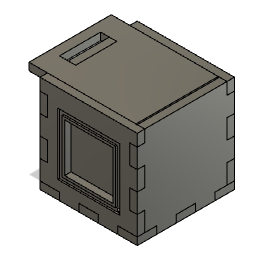
CNC Safe Box v15 (Autodesk Fusion 360 design; units mm, degrees)
Autodesk Fusion 360 part; units mm, degrees
box "BoxPrimitive1" add length 300 width 300 height 23 placed x (0, 0, -1) y (-1, 0, 0) z (0, 1, 0) at (300, 0, 0) makes body 1
sketch "Sketch3" plane through (0, 0, 0) normal (0, 0, 1) x (1, 0, 0)
  line L0 (0, 23) -> (0, 0)
  line L1 (0, 0) -> (300, 0)
  line L2 (300, 0) -> (300, 23)
  line L3 (300, 23) -> (0, 23)
  line L4 (60, 23) -> (120, 23)
  line L5 (120, 23) -> (120, 0)
  line L6 (120, 0) -> (60, 0)
  line L7 (60, 0) -> (60, 23)
  dimension "d20" = 60
  dimension "d21" = 23
  dimension "d22" = 60
  constraint horizontal L4
  constraint vertical L5
  constraint horizontal L6
  constraint vertical L7
  constraint coincident L3 L4.start
  measures "d20" distance of L4.start L4.end
  measures "d21" distance of L4.start L6.end
  measures "d22" distance of L0.start L4.start
extrude "Extrude1" cut sketch "Sketch3" against normal blind 23 contours L1 L3 L4 L5 L6 L7 bodies 1
pattern_linear "R-Pattern1" count 2 spacing 120 along (1, 0, 0) of 3 faces at (60, 7.6667, -7.6667) (80, 7.6667, -23) (120, 15.3333, -7.6667) on bodies 1
sketch "Sketch4" plane through (0, 0, 0) normal (-1, 0, 0) x (0, 0, 1)
  line L0 (-300, 23) -> (-300, 0)
  line L1 (-300, 0) -> (0, 0)
  line L2 (0, 0) -> (0, 23)
  line L3 (0, 23) -> (-300, 23)
  line L4 (-60, 23) -> (-120, 23)
  line L5 (-120, 23) -> (-120, 0)
  line L6 (-120, 0) -> (-60, 0)
  line L7 (-60, 0) -> (-60, 23)
  dimension "d29" = 60
  dimension "d30" = 23
  dimension "d31" = 60
  constraint horizontal L4
  constraint vertical L5
  constraint horizontal L6
  constraint vertical L7
  constraint coincident L3 L4.start
  measures "d29" distance of L4.start L4.end
  measures "d30" distance of L4.start L6.end
  measures "d31" distance of L2.end L4.start
extrude "Extrude2" cut sketch "Sketch4" against normal blind 23 contours L1 L3 L4 L5 L6 L7 bodies 1
pattern_linear "R-Pattern2" count 2 spacing 120 along (0, 0, -1) of 3 faces at (7.6667, 7.6667, -60) (23, 15.3333, -80) (7.6667, 15.3333, -120) on bodies 1
sketch "Sketch5" plane through (0, 0, 0) normal (0, 0, 1) x (1, 0, 0)
  line L0 (0, 0) -> (300, 0)
  line L1 (300, 0) -> (300, 300)
  line L2 (300, 300) -> (0, 300)
  line L3 (0, 300) -> (0, 0)
  dimension "d38" = 300
  dimension "d39" = 300
  constraint horizontal L0
  constraint vertical L1
  constraint horizontal L2
  constraint vertical L3
  constraint coincident L0.start L3.end
  measures "d38" distance of L0.start L0.end
  measures "d39" distance of L0.start L2.end
extrude "Extrude3" add sketch "Sketch5" against normal blind 23 separate body makes body 2
combine "Combine1" operation cut target body 2 tool bodies 1 keep tools
sketch "Sketch6" plane through (0, 0, 0) normal (-1, 0, 0) x (0, 0, 1)
  line L0 (-23, 23) -> (0, 23)
  line L1 (0, 23) -> (0, 300)
  line L2 (0, 300) -> (-23, 300)
  line L3 (-23, 300) -> (-23, 23)
  line L4 (-23, 83) -> (0, 83)
  line L5 (0, 83) -> (0, 143)
  line L6 (0, 143) -> (-23, 143)
  line L7 (-23, 143) -> (-23, 83)
  dimension "d42" = 23
  dimension "d43" = 60
  dimension "d44" = 60
  constraint horizontal L4
  constraint vertical L5
  constraint horizontal L6
  constraint vertical L7
  constraint coincident L3 L4.start
  measures "d42" distance of L4.start L4.end
  measures "d43" distance of L4.start L6.end
  measures "d44" distance of L0.start L4.start
extrude "Extrude4" cut sketch "Sketch6" against normal blind 23 contours L1 L3 L4 L5 L6 L7 bodies 2
pattern_linear "R-Pattern3" count 2 spacing 120 along (0, 1, 0) of 3 faces at (7.6667, 83, -15.3333) (23, 103, -15.3333) (7.6667, 143, -7.6667) on bodies 2
sketch "Sketch7" plane through (0, 0, 0) normal (1, 0, 0) x (0, 0, -1)
  line L0 (0, 0) -> (300, 0)
  line L1 (300, 0) -> (300, 300)
  line L2 (300, 300) -> (0, 300)
  line L3 (0, 300) -> (0, 0)
  dimension "d54" = 300
  dimension "d55" = 300
  constraint horizontal L0
  constraint vertical L1
  constraint horizontal L2
  constraint vertical L3
  constraint coincident L0.start L3.end
  measures "d54" distance of L0.start L0.end
  measures "d55" distance of L0.start L2.end
extrude "Extrude6" add sketch "Sketch7" along normal blind 23 separate body makes body 3
combine "Combine3" operation cut target body 3 tool bodies 2 1 keep tools
extrude "Extrude7" add 1 faces at (23, 175.3333, -167.6667) along direction (-1, 0, 0) blind 23 from surface at -277 separate body on bodies 3 makes body 4
combine "Combine4" operation cut target body 1 tool bodies 4 keep tools
combine "Combine5" operation cut target body 2 tool bodies 4 keep tools
extrude "Extrude10" add 1 faces at (140, 103, -23) along direction (0, 0, 1) blind 23 from surface at -277 separate body on bodies 2 makes body 5
combine "Combine7" operation cut target body 3 tool bodies 5 keep tools
combine "Combine8" operation cut target body 1 tool bodies 5 keep tools
combine "Combine9" operation cut target body 4 tool bodies 5 keep tools
sketch "Sketch9" plane through (0, 300, 0) normal (0, 1, 0) x (-1, 0, 0)
  line L0 (-23, -277) -> (0, -277)
  line L1 (0, -277) -> (0, -23)
  line L2 (0, -23) -> (-23, -23)
  line L3 (-23, -23) -> (-23, -277)
  line L4 (-23, -23) -> (-273, -23)
  line L5 (-273, -23) -> (-273, -277)
  line L6 (-273, -277) -> (-23, -277)
  line L7 (-23, -277) -> (-23, -23)
  dimension "d75" = 250
  dimension "d76" = 254
  constraint horizontal L4
  constraint vertical L5
  constraint horizontal L6
  constraint vertical L7
  constraint coincident L2.end L3.start
  measures "d75" distance of L2.end L4.end
  measures "d76" distance of L2.end L0.start
extrude "Extrude11" add sketch "Sketch9" against normal blind 23 separate body contours L3 L4 L5 L6 L7 makes body 6
sketch "Sketch14" plane through (23, 0, 0) normal (-1, 0, 0) x (0, 0, 1)
  line L0 (-23, 300) -> (-277, 300)
  line L1 (-277, 300) -> (-277, 277)
  line L2 (-277, 277) -> (-23, 277)
  line L3 (-23, 277) -> (-23, 300)
  line L4 (-87, 300) -> (-214, 300)
  line L5 (-214, 300) -> (-214, 277)
  line L6 (-214, 277) -> (-87, 277)
  line L7 (-87, 277) -> (-87, 300)
  line L8 (-87, 300) -> (-214, 277) construction
  line L9 (-214, 300) -> (-87, 277) construction
  point P0 (-150.5, 288.5)
  dimension "d146" = 127
  dimension "d147" = 23
  constraint horizontal L4
  constraint perpendicular L4 L5
  constraint parallel L4 L6
  constraint parallel L5 L7
  constraint coincident L8 P0
  constraint coincident L9 P0
  measures "d146" distance of L5.end L6.end
  measures "d147" distance of L4.end L5.end
extrude "Extrude22" add sketch "Sketch14" along normal blind 80 contours L0 L2 L3 L7 | L0 L1 L2 L5 bodies 6
extrude "Extrude23" add 1 faces at (23, 292.3333, -129.3333) along direction (1, 0, 0) blind 30 from surface at -80 on bodies 6 bodies 6
combine "Combine11" operation cut target body 3 tool bodies 6 keep tools
sketch "Sketch15" plane through (0, 0, 0) normal (0, 0, 1) x (1, 0, 0)
  line L0 (300, 300) -> (0, 300)
  line L1 (0, 300) -> (0, 263)
  line L2 (0, 263) -> (23, 263)
  line L3 (23, 263) -> (23, 203)
  line L4 (23, 203) -> (0, 203)
  line L5 (0, 203) -> (0, 143)
  line L6 (0, 143) -> (23, 143)
  line L7 (23, 143) -> (23, 83)
  line L8 (23, 83) -> (0, 83)
  line L9 (0, 83) -> (0, 23)
  line L10 (0, 23) -> (60, 23)
  line L11 (60, 23) -> (60, 0)
  line L12 (60, 0) -> (120, 0)
  line L13 (120, 0) -> (120, 23)
  line L14 (120, 23) -> (180, 23)
  line L15 (180, 23) -> (180, 0)
  line L16 (180, 0) -> (240, 0)
  line L17 (240, 0) -> (240, 23)
  line L18 (240, 23) -> (300, 23)
  line L19 (300, 23) -> (300, 83)
  line L20 (300, 83) -> (277, 83)
  line L21 (277, 83) -> (277, 143)
  line L22 (277, 143) -> (300, 143)
  line L23 (300, 143) -> (300, 203)
  line L24 (300, 203) -> (277, 203)
  line L25 (277, 203) -> (277, 263)
  line L26 (277, 263) -> (300, 263)
  line L27 (300, 263) -> (300, 300)
  line L28 (76, 75) -> (225, 75)
  line L29 (225, 75) -> (225, 224)
  line L30 (225, 224) -> (76, 224)
  line L31 (76, 224) -> (76, 75)
  line L32 (76, 75) -> (225, 224) construction
  line L33 (225, 75) -> (76, 224) construction
  line L34 (233, 232) -> (68, 232)
  line L35 (68, 232) -> (68, 67)
  line L36 (68, 67) -> (233, 67)
  line L37 (233, 67) -> (233, 232)
  line L38 (246, 245) -> (55, 245)
  line L39 (55, 245) -> (55, 54)
  line L40 (55, 54) -> (246, 54)
  line L41 (246, 54) -> (246, 245)
  circle A0 centre (238.9878, 61.5455) radius 5
  point P0 (150.5, 149.5)
  dimension "d133" = 149
  dimension "d134" = 149
  dimension "d135" = 8
  dimension "d136" = 21
  dimension "d138" = 10
  constraint horizontal L28
  constraint perpendicular L28 L29
  constraint parallel L28 L30
  constraint parallel L29 L31
  constraint coincident L32 P0
  constraint coincident L33 P0
  measures "d133" distance of L29.end L30.end
  measures "d134" distance of L28.end L29.end
  measures "d138" diameter of A0
extrude "Extrude24" cut sketch "Sketch15" against normal blind 20 contours L28 L29 L30 L31 bodies 2
extrude "Extrude25" cut sketch "Sketch15" against normal blind 5 contours L38 L39 L40 L41 bodies 2
extrude "Extrude26" cut sketch "Sketch15" against normal blind 23 contours A0 bodies 2
sketch "Sketch16" plane through (300, 0, 0) normal (1, 0, 0) x (0, 0, -1)
  line L0 (277, 23) -> (277, 83)
  line L1 (277, 83) -> (300, 83)
  line L2 (300, 83) -> (300, 143)
  line L3 (300, 143) -> (277, 143)
  line L4 (277, 143) -> (277, 203)
  line L5 (277, 203) -> (300, 203)
  line L6 (300, 203) -> (300, 263)
  line L7 (300, 263) -> (277, 263)
  line L8 (277, 263) -> (277, 300)
  line L9 (277, 300) -> (23, 300)
  line L10 (23, 300) -> (23, 263)
  line L11 (23, 263) -> (0, 263)
  line L12 (0, 263) -> (0, 203)
  line L13 (0, 203) -> (23, 203)
  line L14 (23, 203) -> (23, 143)
  line L15 (23, 143) -> (0, 143)
  line L16 (0, 143) -> (0, 83)
  line L17 (0, 83) -> (23, 83)
  line L18 (23, 83) -> (23, 23)
  line L19 (23, 23) -> (60, 23)
  line L20 (60, 23) -> (60, 0)
  line L21 (60, 0) -> (120, 0)
  line L22 (120, 0) -> (120, 23)
  line L23 (120, 23) -> (180, 23)
  line L24 (180, 23) -> (180, 0)
  line L25 (180, 0) -> (240, 0)
  line L26 (240, 0) -> (240, 23)
  line L27 (240, 23) -> (277, 23)
sketch "Sketch17" plane through (0, 0, 0) normal (-1, 0, 0) x (0, 0, 1)
  line L0 (-23, 277) -> (-87, 277)
  line L1 (-87, 277) -> (-87, 300)
  line L2 (-87, 300) -> (-214, 300)
  line L3 (-214, 300) -> (-214, 277)
  line L4 (-214, 277) -> (-277, 277)
  line L5 (-277, 277) -> (-277, 263)
  line L6 (-277, 263) -> (-300, 263)
  line L7 (-300, 263) -> (-300, 203)
  line L8 (-300, 203) -> (-277, 203)
  line L9 (-277, 203) -> (-277, 143)
  line L10 (-277, 143) -> (-300, 143)
  line L11 (-300, 143) -> (-300, 83)
  line L12 (-300, 83) -> (-277, 83)
  line L13 (-277, 83) -> (-277, 23)
  line L14 (-277, 23) -> (-240, 23)
  line L15 (-240, 23) -> (-240, 0)
  line L16 (-240, 0) -> (-180, 0)
  line L17 (-180, 0) -> (-180, 23)
  line L18 (-180, 23) -> (-120, 23)
  line L19 (-120, 23) -> (-120, 0)
  line L20 (-120, 0) -> (-60, 0)
  line L21 (-60, 0) -> (-60, 23)
  line L22 (-60, 23) -> (-23, 23)
  line L23 (-23, 23) -> (-23, 83)
  line L24 (-23, 83) -> (0, 83)
  line L25 (0, 83) -> (0, 143)
  line L26 (0, 143) -> (-23, 143)
  line L27 (-23, 143) -> (-23, 203)
  line L28 (-23, 203) -> (0, 203)
  line L29 (0, 203) -> (0, 263)
  line L30 (0, 263) -> (-23, 263)
  line L31 (-23, 263) -> (-23, 277)
sketch "Sketch18" plane through (0, 0, -300) normal (0, 0, -1) x (-1, 0, 0)
  line L0 (-300, 263) -> (-277, 263)
  line L1 (-277, 263) -> (-277, 203)
  line L2 (-277, 203) -> (-300, 203)
  line L3 (-300, 203) -> (-300, 143)
  line L4 (-300, 143) -> (-277, 143)
  line L5 (-277, 143) -> (-277, 83)
  line L6 (-277, 83) -> (-300, 83)
  line L7 (-300, 83) -> (-300, 23)
  line L8 (-300, 23) -> (-240, 23)
  line L9 (-240, 23) -> (-240, 0)
  line L10 (-240, 0) -> (-180, 0)
  line L11 (-180, 0) -> (-180, 23)
  line L12 (-180, 23) -> (-120, 23)
  line L13 (-120, 23) -> (-120, 0)
  line L14 (-120, 0) -> (-60, 0)
  line L15 (-60, 0) -> (-60, 23)
  line L16 (-60, 23) -> (0, 23)
  line L17 (0, 23) -> (0, 83)
  line L18 (0, 83) -> (-23, 83)
  line L19 (-23, 83) -> (-23, 143)
  line L20 (-23, 143) -> (0, 143)
  line L21 (0, 143) -> (0, 203)
  line L22 (0, 203) -> (-23, 203)
  line L23 (-23, 203) -> (-23, 263)
  line L24 (-23, 263) -> (0, 263)
  line L25 (0, 263) -> (0, 300)
  line L26 (0, 300) -> (-300, 300)
  line L27 (-300, 300) -> (-300, 263)
sketch "Sketch19" plane through (0, 0, 0) normal (0, -1, 0) x (1, 0, 0)
  line L0 (240, -277) -> (240, -300)
  line L1 (240, -300) -> (300, -300)
  line L2 (300, -300) -> (300, -240)
  line L3 (300, -240) -> (277, -240)
  line L4 (277, -240) -> (277, -180)
  line L5 (277, -180) -> (300, -180)
  line L6 (300, -180) -> (300, -120)
  line L7 (300, -120) -> (277, -120)
  line L8 (277, -120) -> (277, -60)
  line L9 (277, -60) -> (300, -60)
  line L10 (300, -60) -> (300, 0)
  line L11 (300, 0) -> (240, 0)
  line L12 (240, 0) -> (240, -23)
  line L13 (240, -23) -> (180, -23)
  line L14 (180, -23) -> (180, 0)
  line L15 (180, 0) -> (120, 0)
  line L16 (120, 0) -> (120, -23)
  line L17 (120, -23) -> (60, -23)
  line L18 (60, -23) -> (60, 0)
  line L19 (60, 0) -> (0, 0)
  line L20 (0, 0) -> (0, -60)
  line L21 (0, -60) -> (23, -60)
  line L22 (23, -60) -> (23, -120)
  line L23 (23, -120) -> (0, -120)
  line L24 (0, -120) -> (0, -180)
  line L25 (0, -180) -> (23, -180)
  line L26 (23, -180) -> (23, -240)
  line L27 (23, -240) -> (0, -240)
  line L28 (0, -240) -> (0, -300)
  line L29 (0, -300) -> (60, -300)
  line L30 (60, -300) -> (60, -277)
  line L31 (60, -277) -> (120, -277)
  line L32 (120, -277) -> (120, -300)
  line L33 (120, -300) -> (180, -300)
  line L34 (180, -300) -> (180, -277)
  line L35 (180, -277) -> (240, -277)
sketch "Sketch20" plane through (0, 300, 0) normal (0, 1, 0) x (-1, 0, 0)
  line L0 (27, -214) -> (-23, -214)
  line L1 (-23, -214) -> (-23, -87)
  line L2 (-23, -87) -> (27, -87)
  line L3 (27, -87) -> (27, -214)
  line L4 (57, -277) -> (57, -23)
  line L5 (57, -23) -> (-273, -23)
  line L6 (-273, -23) -> (-273, -277)
  line L7 (-273, -277) -> (57, -277)
equation "Length = 300 mm"
equation "Width = 300 mm"
equation "Height = 300 mm"
equation "Thickness = 23 mm"
equation "LSTab = 2"
equation "WSTab = 2"
equation "HSTab = 2"
equation "LTabForm = Length / ( ( LSTab * 2 ) + 1 )"
equation "WTabForm = Width / ( ( WSTab * 2 ) + 1 )"
equation "HTabForm = Height / ( ( HSTab * 2 ) + 1 )"
equation "LPattForm = ( Length - ( LTabForm * 3 ) )"
equation "WPattForm = ( Width - ( WTabForm * 3 ) )"
equation "HPattForm = ( Height - ( HTabForm * 3 ) )"
equation "d15 = Width"
equation "d16 = Length"
equation "d17 = Thickness"
equation "d20 = LTabForm"
equation "d21 = Thickness"
equation "d22 = LTabForm"
equation "d23 = -Thickness"
equation "d25 = LSTab"
equation "d27 = -LPattForm"
equation "d29 = WTabForm"
equation "d30 = Thickness"
equation "d31 = WTabForm"
equation "d32 = -Thickness"
equation "d34 = WSTab"
equation "d36 = -WPattForm"
equation "d38 = Length"
equation "d39 = Height"
equation "d40 = -Thickness"
equation "d42 = Thickness"
equation "d43 = HTabForm"
equation "d44 = HTabForm"
equation "d45 = -Thickness"
equation "d47 = HSTab"
equation "d49 = -HPattForm"
equation "d54 = Width"
equation "d55 = Height"
equation "d56 = Thickness"
equation "d59 = -Thickness"
equation "d73 = -Thickness"
equation "d75 = LTop"
equation "d76 = WTop"
equation "d78 = -Thickness"
equation "Whandle = 80 mm"
equation "FHandle = 10 mm"
equation "LPuzzle = 149 mm"
equation "WPuzzle = 149 mm"
equation "DPuzzle = Thickness - 3 mm"
equation "OLeds = 21 mm" comment "Offset for leds"
equation "DLeds = 5 mm"
equation "LTop = 250 mm"
equation "WTop = 254 mm"
equation "d127 = Whandle"
equation "d130 = -Thickness - 7 mm"
equation "d133 = LPuzzle"
equation "d134 = WPuzzle"
equation "d136 = OLeds"
equation "DiameterLeds = 10 mm"
equation "d138 = DiameterLeds"
equation "d139 = -DPuzzle"
equation "d141 = -DLeds"
equation "d143 = -Thickness"
equation "d146 = WTop / 2"
equation "d147 = Thickness"
